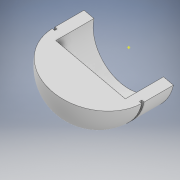
# Autodesk Inventor part: HoseConnector
Saved by Autodesk Inventor 2020.4 (Build 244396010, 396A)
## iProperties
Created: 2022-09-10
Part Number: HoseConnector
Material: Generic
Document SubType Name: Modeling
Designer: Val
Density: 1 g/cm^3
Appearance: Default
Author: Val
Autodesk Inventor part; units mm, degrees
ref_plane "YZ Plane" through (0, 0, 0) normal (1, 0, 0) x (0, 1, 0)
ref_plane "XZ Plane" through (0, 0, 0) normal (0, 1, 0) x (-1, 0, 0)
ref_plane "XY Plane" through (0, 0, 0) normal (0, 0, 1) x (1, 0, 0)
sketch "Base" plane through (0, 0, 0) normal (0, 0, 1) x (1, 0, 0)
  circle A0 centre (0, 0) radius 38.1
  dimension "d0" = 76.2
  constraints: 1 centre point, 1 coincident
  measures "d0" diameter of A0
extrude "BaseFeature" add sketch "Base" along normal blind 63.5
fillet "BaseFilletsFeature" radius 38.1 1 edges at (-38.1, 0, 63.5)
split "HalfCutFeature" plane through (-274.3569, 62.0713, -19.3818) removes the side toward (0.2206659, 0.9753495, 0)
ref_plane "HalfCut" through (-274.3569, 62.0713, -19.3818) normal (-0.2206659, -0.9753495, 0) x (-0.9357661, 0.2117104, -0.2819939)
ref_plane "RidgePlane" through (0, 0, 25.4) normal (0, 0, -1) x (-1, 0, 0)
sketch "RidgeProfile" plane through (0, 0, 25.4) normal (0, 0, -1) x (-1, 0, 0)
  circle A0 centre (0, 0) radius 36.1
  arc A1 (-37.1608, -8.4074) -> (37.1608, 8.4074) centre (0, 0) ccw projected
  arc A2 (-37.1608, -8.4074) -> (37.1608, 8.4074) centre (0, 0) ccw projected
  circle A3 centre (0, 0) radius 38.1
  point P0 (-37.1608, -8.4074)
  dimension "d5" = 2
  constraints: 2 coincident, 1 centre point, 3 other
extrude "RidgeCutFeature" cut sketch "RidgeProfile" along normal mid plane 2
sketch "InsideCutProfile" plane through (0, 0, 0) normal (0, 0, -1) x (-1, 0, 0)
  line L0 (37.1608, 8.4074) -> (-37.1608, -8.4074) projected
  arc A0 (-37.1608, -8.4074) -> (37.1608, 8.4074) centre (0, 0) ccw projected
  line L1 (-29.5755, 1.9807) -> (25.8427, 14.5187)
  arc A1 (-29.5755, 1.9807) -> (25.8427, 14.5187) centre (0, 0) ccw
  line L2 (-36.6699, -7.6367) -> (36.386, 8.8916) construction
  arc A2 (-36.6699, -7.6367) -> (36.386, 8.8916) centre (0, 0) ccw
  line L3 (25.8427, 14.5187) -> (27.7091, 6.269)
  line L4 (-37.148, -8.4045) -> (37.148, 8.4045) projected
  line L5 (-29.5755, 1.9807) -> (-27.7091, -6.269)
  line L6 (37.1608, 8.4074) -> (-37.1608, -8.4074) projected
  line L7 (27.7091, 6.269) -> (-27.7091, -6.269)
  point P0 (27.5672, 6.8964)
  point P1 (-27.8511, -5.6415)
  point P2 (-27.7091, -6.269)
  dimension "d13" = 8.4582
  constraints: 10 end point, 4 point on circle, 2 centre point, 2 perpendicular, 2 point on line, 1 collinear, 2 other
  measures "d13" radial gap between concentric circles of A0 A1
extrude "InsideCutFeature" cut sketch "InsideCutProfile" against normal blind 31.75 contours A1 L0 | L0 L3 A1 | L0 L5 L1 L3 | A1 L5 L0
body "Solid1"
